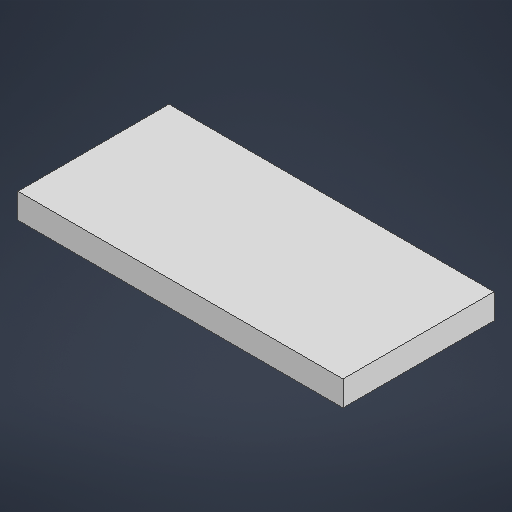
# Autodesk Inventor part: Bridge Plate
Saved by Autodesk Inventor 2026.3 (Build 303398000, 398)
## iProperties
Created: 2026-06-29
Part Number: Bridge Plate
Material: Generic
Document SubType Name: Modeling
Designer: Inigo Greenall
Density: 1 g/cm^3
Appearance: Default
Author: Inigo Greenall
Autodesk Inventor part; units mm, degrees
ref_plane "YZ Plane" through (0, 0, 0) normal (1, 0, 0) x (0, 1, 0)
ref_plane "XZ Plane" through (0, 0, 0) normal (0, 1, 0) x (-1, 0, 0)
ref_plane "XY Plane" through (0, 0, 0) normal (0, 0, 1) x (1, 0, 0)
sketch "Sketch1" plane through (0, 0, 0) normal (0, 1, 0) x (-1, 0, 0)
  line L0 (64.9, 30.15) -> (-64.9, 30.15)
  line L1 (-64.9, 30.15) -> (-64.9, -30.15)
  line L2 (-64.9, -30.15) -> (64.9, -30.15)
  line L3 (64.9, -30.15) -> (64.9, 30.15)
  point P0 (0, 0)
  point P1 (64.9, 0)
  point P2 (0, 30.15)
  dimension "d0" = 60.3
  dimension "d1" = 129.8
  constraints: 8 end point, 2 midpoint, 2 parallel, 1 horizontal, 1 horizontal alignment, 1 perpendicular, 1 vertical alignment
  measures "d0" distance of L2.end L0.start
  measures "d1" distance of L1.end L2.end
extrude "Extrusion2" add sketch "Sketch1" along normal blind 10
body "Solid2"
